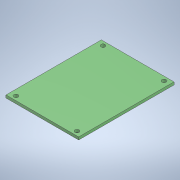
# Autodesk Inventor part: Mock Module PCB
Saved by Autodesk Inventor 2022 (Build 260153000, 153)
## iProperties
Created: 2021-07-19
Part Number: Mock Module PCB
Material: Generic
Document SubType Name: Modeling
Designer: Caleb
Density: 1 g/cm^3
Appearance: Default
Author: Caleb
Autodesk Inventor part; units mm, degrees
ref_plane "YZ Plane" through (0, 0, 0) normal (1, 0, 0) x (0, 1, 0)
ref_plane "XZ Plane" through (0, 0, 0) normal (0, 1, 0) x (-1, 0, 0)
ref_plane "XY Plane" through (0, 0, 0) normal (0, 0, 1) x (1, 0, 0)
sketch "Sketch1" plane through (0, 0, 0) normal (0, 1, 0) x (-1, 0, 0)
  line L0 (-21.5, 28.2) -> (21.5, 28.2)
  line L1 (21.5, 28.2) -> (21.5, -28.2)
  line L2 (21.5, -28.2) -> (-21.5, -28.2)
  line L3 (-21.5, -28.2) -> (-21.5, 28.2)
  line L4 (-21.5, 28.2) -> (21.5, -28.2) construction
  line L5 (21.5, 28.2) -> (-21.5, -28.2) construction
  point P0 (0, 0)
  dimension "d0" = 43
  dimension "d1" = 56.4
  constraints: 12 end point, 2 midpoint, 2 parallel, 1 horizontal, 1 perpendicular
  measures "d0" distance of L0.start L0.end
  measures "d1" distance of L0.end L1.end
extrude "Extrusion1" add sketch "Sketch1" along normal blind 1.6
sketch "Sketch2" plane through (0, 1.6, 0) normal (0, 1, 0) x (1, 0, 0)
  point P0 (0, 0)
  point P1 (-18.05, -25.75)
  point P2 (-18.05, 25.75)
  point P3 (18.05, 25.75)
  point P4 (18.05, -25.75)
  dimension "d19" = 36.1
  dimension "d20" = 51.5
  dimension "d21" = 25.75
  dimension "d22" = 18.05
  constraints: 2 horizontal alignment, 2 vertical alignment
  measures "d19" distance of point (18.05, 25.75) point (-18.05, 25.75)
  measures "d20" distance of point (-18.05, -25.75) point (-18.05, 25.75)
  measures "d21" vertical distance of point (0, 0) point (-18.05, 25.75)
  measures "d22" horizontal distance of point (0, 0) point (18.05, 25.75)
hole "Hole1" at (-18.05, 1.6, 25.75) at (-18.05, 1.6, -25.75) at (18.05, 1.6, -25.75) at (18.05, 1.6, 25.75) direction (0, -1, 0) diameter 2.5 end through all
sketch "Sketch4" plane through (0, 0, 0) normal (0, -1, 0) x (1, 0, 0)
  line L0 (10.5954, -26.3152) -> (-11.3358, -26.3152) construction
  line L1 (-11.3358, -26.3152) -> (-11.3358, -23.0671) construction
  line L2 (-11.3358, -23.0671) -> (10.5954, -23.0671) construction
  line L3 (10.5954, -23.0671) -> (10.5954, -26.3152) construction
  line L4 (7.6734, -23.1313) -> (8.0785, -23.1313)
  line L5 (8.0785, -23.1313) -> (8.0785, -25.7569)
  line L6 (8.0785, -25.7569) -> (8.8738, -23.9711)
  line L7 (8.8738, -23.9711) -> (9.1208, -23.9711)
  line L8 (9.1208, -23.9711) -> (9.9088, -25.7569)
  line L9 (9.9088, -25.7569) -> (9.9088, -23.1313)
  line L10 (9.9088, -23.1313) -> (10.2867, -23.1313)
  line L11 (10.2867, -23.1313) -> (10.2867, -26.1793)
  line L12 (10.2867, -26.1793) -> (9.7334, -26.1793)
  line L13 (9.7334, -26.1793) -> (8.9726, -24.4824)
  line L14 (8.9726, -24.4824) -> (8.2366, -26.1793)
  line L15 (8.2366, -26.1793) -> (7.6734, -26.1793)
  line L16 (7.6734, -26.1793) -> (7.6734, -23.1313)
  spline S0 degree 2 poles (5.2059, -24.2749) (5.2059, -23.6969) (5.7616, -23.0671) (6.226, -23.0671) knots 0 0 0 1 2 2 2
  spline S1 degree 2 poles (6.226, -23.0671) (6.7027, -23.0671) (7.2486, -23.7167) (7.2486, -24.2749) knots 0 0 0 1 2 2 2
  spline S2 degree 2 poles (7.2486, -24.2749) (7.2486, -24.848) (6.6854, -25.4828) (6.226, -25.4828) knots 0 0 0 1 2 2 2
  spline S3 degree 2 poles (6.226, -25.4828) (5.7616, -25.4828) (5.2059, -24.8504) (5.2059, -24.2749) knots 0 0 0 1 2 2 2
  spline S4 degree 2 poles (5.6035, -24.2749) (5.6035, -24.7195) (5.9271, -25.1518) (6.226, -25.1518) knots 0 0 0 1 2 2 2
  spline S5 degree 2 poles (6.226, -25.1518) (6.5249, -25.1518) (6.8509, -24.7195) (6.8509, -24.2749) knots 0 0 0 1 2 2 2
  spline S6 degree 2 poles (6.8509, -24.2749) (6.8509, -23.8427) (6.5249, -23.3981) (6.226, -23.3981) knots 0 0 0 1 2 2 2
  spline S7 degree 2 poles (6.226, -23.3981) (5.9296, -23.3981) (5.6035, -23.8353) (5.6035, -24.2749) knots 0 0 0 1 2 2 2
  line L17 (3.052, -23.1313) -> (3.4373, -23.1313)
  line L18 (3.4373, -23.1313) -> (3.4373, -23.3635)
  spline S8 degree 2 poles (3.4373, -23.3635) (3.5263, -23.2894) (3.6572, -23.1906) (3.7461, -23.1486) knots 0 0 0 1 2 2 2
  spline S9 degree 2 poles (3.7461, -23.1486) (3.8276, -23.1091) (4.003, -23.0671) (4.1191, -23.0671) knots 0 0 0 1 2 2 2
  spline S10 degree 2 poles (4.1191, -23.0671) (4.3068, -23.0671) (4.6229, -23.2227) (4.7341, -23.3734) knots 0 0 0 1 2 2 2
  spline S11 degree 2 poles (4.7341, -23.3734) (4.8452, -23.524) (4.9687, -23.9687) (4.9687, -24.2576) knots 0 0 0 1 2 2 2
  spline S12 degree 2 poles (4.9687, -24.2576) (4.9687, -24.559) (4.8131, -24.9986) (4.6773, -25.1641) knots 0 0 0 1 2 2 2
  spline S13 degree 2 poles (4.6773, -25.1641) (4.5513, -25.3123) (4.1981, -25.4828) (4.003, -25.4828) knots 0 0 0 1 2 2 2
  spline S14 degree 2 poles (4.003, -25.4828) (3.8325, -25.4828) (3.5781, -25.4062) (3.4373, -25.3272) knots 0 0 0 1 2 2 2
  line L19 (3.4373, -25.3272) -> (3.4373, -26.3152)
  line L20 (3.4373, -26.3152) -> (3.052, -26.3152)
  line L21 (3.052, -26.3152) -> (3.052, -23.1313)
  line L22 (3.4373, -23.6871) -> (3.4373, -25.0085)
  spline S15 degree 2 poles (3.4373, -25.0085) (3.5806, -25.0777) (3.8078, -25.1296) (3.9387, -25.1296) knots 0 0 0 1 2 2 2
  spline S16 degree 2 poles (3.9387, -25.1296) (4.2351, -25.1296) (4.5711, -24.685) (4.5711, -24.2651) knots 0 0 0 1 2 2 2
  spline S17 degree 2 poles (4.5711, -24.2651) (4.5711, -23.86) (4.3142, -23.4327) (4.0301, -23.4327) knots 0 0 0 1 2 2 2
  spline S18 degree 2 poles (4.0301, -23.4327) (3.8795, -23.4327) (3.5732, -23.571) (3.4373, -23.6871) knots 0 0 0 1 2 2 2
  line L23 (0.7154, -23.1313) -> (1.1007, -23.1313)
  line L24 (1.1007, -23.1313) -> (1.1007, -23.3833)
  spline S19 degree 2 poles (1.1007, -23.3833) (1.2785, -23.2276) (1.5972, -23.0671) (1.7948, -23.0671) knots 0 0 0 1 2 2 2
  spline S20 degree 2 poles (1.7948, -23.0671) (1.943, -23.0671) (2.2073, -23.1659) (2.3036, -23.2721) knots 0 0 0 1 2 2 2
  spline S21 degree 2 poles (2.3036, -23.2721) (2.4024, -23.3783) (2.5111, -23.7019) (2.5111, -23.9341) knots 0 0 0 1 2 2 2
  line L25 (2.5111, -23.9341) -> (2.5111, -25.4186)
  line L26 (2.5111, -25.4186) -> (2.1258, -25.4186)
  line L27 (2.1258, -25.4186) -> (2.1258, -24.1144)
  spline S22 degree 2 poles (2.1258, -24.1144) (2.1258, -23.9316) (2.0986, -23.692) (2.0517, -23.6031) knots 0 0 0 1 2 2 2
  spline S23 degree 2 poles (2.0517, -23.6031) (2.0047, -23.5142) (1.8442, -23.4327) (1.6935, -23.4327) knots 0 0 0 1 2 2 2
  spline S24 degree 2 poles (1.6935, -23.4327) (1.5527, -23.4327) (1.2341, -23.5932) (1.1007, -23.7093) knots 0 0 0 1 2 2 2
  line L28 (1.1007, -23.7093) -> (1.1007, -25.4186)
  line L29 (1.1007, -25.4186) -> (0.7154, -25.4186)
  line L30 (0.7154, -25.4186) -> (0.7154, -23.1313)
  line L31 (-0.2356, -23.1313) -> (0.1497, -23.1313)
  line L32 (0.1497, -23.1313) -> (0.1497, -26.3152)
  line L33 (0.1497, -26.3152) -> (-0.2356, -26.3152)
  line L34 (-0.2356, -26.3152) -> (-0.2356, -23.1313)
  spline S25 degree 2 poles (-1.7942, -23.0794) (-1.2458, -23.0794) (-0.6431, -23.6945) (-0.6431, -24.2626) knots 0 0 0 1 2 2 2
  spline S26 degree 2 poles (-0.6431, -24.2626) (-0.6431, -24.8208) (-1.2285, -25.4828) (-1.7003, -25.4828) knots 0 0 0 1 2 2 2
  spline S27 degree 2 poles (-1.7003, -25.4828) (-1.9127, -25.4828) (-2.2412, -25.3593) (-2.3623, -25.2284) knots 0 0 0 1 2 2 2
  spline S28 degree 2 poles (-2.3623, -25.2284) (-2.4858, -25.0974) (-2.6167, -24.7195) (-2.6167, -24.4454) knots 0 0 0 1 2 2 2
  line L35 (-2.6167, -24.4454) -> (-2.6167, -24.2354)
  line L36 (-2.6167, -24.2354) -> (-1.0334, -24.2354)
  spline S29 degree 2 poles (-1.0334, -24.2354) (-1.0334, -23.8377) (-1.4335, -23.4154) (-1.7892, -23.4154) knots 0 0 0 1 2 2 2
  spline S30 degree 2 poles (-1.7892, -23.4154) (-1.9152, -23.4154) (-2.1597, -23.4722) (-2.2585, -23.5166) knots 0 0 0 1 2 2 2
  spline S31 degree 2 poles (-2.2585, -23.5166) (-2.3623, -23.566) (-2.5055, -23.6525) (-2.5525, -23.692) knots 0 0 0 1 2 2 2
  line L37 (-2.5525, -23.692) -> (-2.5747, -23.692)
  line L38 (-2.5747, -23.692) -> (-2.5747, -23.2721)
  spline S32 degree 2 poles (-2.5747, -23.2721) (-2.508, -23.2449) (-2.3055, -23.1659) (-2.2264, -23.1437) knots 0 0 0 1 2 2 2
  spline S33 degree 2 poles (-2.2264, -23.1437) (-2.1153, -23.1116) (-1.9325, -23.0794) (-1.7942, -23.0794) knots 0 0 0 1 2 2 2
  spline S34 degree 2 poles (-2.2412, -24.5293) (-2.2363, -24.685) (-2.1721, -24.9122) (-2.1103, -24.9888) knots 0 0 0 1 2 2 2
  spline S35 degree 2 poles (-2.1103, -24.9888) (-2.0436, -25.0752) (-1.8337, -25.1666) (-1.6781, -25.1666) knots 0 0 0 1 2 2 2
  spline S36 degree 2 poles (-1.6781, -25.1666) (-1.5249, -25.1666) (-1.31, -25.0752) (-1.2211, -24.9863) knots 0 0 0 1 2 2 2
  spline S37 degree 2 poles (-1.2211, -24.9863) (-1.1347, -24.8949) (-1.0457, -24.6751) (-1.0334, -24.5293) knots 0 0 0 1 2 2 2
  line L39 (-1.0334, -24.5293) -> (-2.2412, -24.5293)
  spline S38 degree 2 poles (-6.2723, -25.2605) (-6.2723, -25.0629) (-6.1315, -24.7072) (-6.0055, -24.5837) knots 0 0 0 1 2 2 2
  spline S39 degree 2 poles (-6.0055, -24.5837) (-5.8475, -24.4281) (-5.4201, -24.2675) (-5.0941, -24.2675) knots 0 0 0 1 2 2 2
  line L40 (-5.0941, -24.2675) -> (-4.7508, -24.2675)
  line L41 (-4.7508, -24.2675) -> (-4.7508, -23.1313)
  line L42 (-4.7508, -23.1313) -> (-4.3457, -23.1313)
  line L43 (-4.3457, -23.1313) -> (-4.3457, -26.1793)
  line L44 (-4.3457, -26.1793) -> (-5.1114, -26.1793)
  spline S40 degree 2 poles (-5.1114, -26.1793) (-5.3831, -26.1793) (-5.7635, -26.0904) (-5.9092, -25.9891) knots 0 0 0 1 2 2 2
  spline S41 degree 2 poles (-5.9092, -25.9891) (-6.0796, -25.873) (-6.2723, -25.5149) (-6.2723, -25.2605) knots 0 0 0 1 2 2 2
  spline S42 degree 2 poles (-5.8499, -25.2481) (-5.8499, -25.4062) (-5.7412, -25.6384) (-5.6301, -25.7125) knots 0 0 0 1 2 2 2
  spline S43 degree 2 poles (-5.6301, -25.7125) (-5.5338, -25.7767) (-5.2769, -25.8286) (-5.0867, -25.8286) knots 0 0 0 1 2 2 2
  line L45 (-5.0867, -25.8286) -> (-4.7508, -25.8286)
  line L46 (-4.7508, -25.8286) -> (-4.7508, -24.6133)
  line L47 (-4.7508, -24.6133) -> (-5.0274, -24.6133)
  spline S44 degree 2 poles (-5.0274, -24.6133) (-5.2744, -24.6133) (-5.5782, -24.6924) (-5.677, -24.7961) knots 0 0 0 1 2 2 2
  spline S45 degree 2 poles (-5.677, -24.7961) (-5.7684, -24.8875) (-5.8499, -25.1024) (-5.8499, -25.2481) knots 0 0 0 1 2 2 2
  spline S46 degree 2 poles (-7.8482, -23.077) (-7.5518, -23.077) (-7.0504, -23.277) (-6.8676, -23.4771) knots 0 0 0 1 2 2 2
  spline S47 degree 2 poles (-6.8676, -23.4771) (-6.6848, -23.6747) (-6.4847, -24.2675) (-6.4847, -24.6528) knots 0 0 0 1 2 2 2
  spline S48 degree 2 poles (-6.4847, -24.6528) (-6.4847, -25.0357) (-6.6799, -25.6038) (-6.8651, -25.8138) knots 0 0 0 1 2 2 2
  spline S49 degree 2 poles (-6.8651, -25.8138) (-7.0479, -26.0188) (-7.5468, -26.2337) (-7.8556, -26.2337) knots 0 0 0 1 2 2 2
  spline S50 degree 2 poles (-7.8556, -26.2337) (-8.0087, -26.2337) (-8.278, -26.1892) (-8.3916, -26.1546) knots 0 0 0 1 2 2 2
  spline S51 degree 2 poles (-8.3916, -26.1546) (-8.4904, -26.1225) (-8.6954, -26.0311) (-8.7967, -25.9768) knots 0 0 0 1 2 2 2
  line L48 (-8.7967, -25.9768) -> (-8.7967, -25.4877)
  line L49 (-8.7967, -25.4877) -> (-8.7645, -25.4877)
  spline S52 degree 2 poles (-8.7645, -25.4877) (-8.7102, -25.5371) (-8.5422, -25.6754) (-8.4212, -25.7421) knots 0 0 0 1 2 2 2
  spline S53 degree 2 poles (-8.4212, -25.7421) (-8.3051, -25.8063) (-8.031, -25.8879) (-7.8531, -25.8879) knots 0 0 0 1 2 2 2
  spline S54 degree 2 poles (-7.8531, -25.8879) (-7.658, -25.8879) (-7.3097, -25.7273) (-7.1788, -25.5742) knots 0 0 0 1 2 2 2
  spline S55 degree 2 poles (-7.1788, -25.5742) (-7.0504, -25.4186) (-6.9071, -24.9468) (-6.9071, -24.6528) knots 0 0 0 1 2 2 2
  spline S56 degree 2 poles (-6.9071, -24.6528) (-6.9071, -24.3392) (-7.0578, -23.8871) (-7.1887, -23.7315) knots 0 0 0 1 2 2 2
  spline S57 degree 2 poles (-7.1887, -23.7315) (-7.3171, -23.5809) (-7.6605, -23.4277) (-7.8531, -23.4277) knots 0 0 0 1 2 2 2
  spline S58 degree 2 poles (-7.8531, -23.4277) (-8.0285, -23.4277) (-8.3274, -23.5142) (-8.4434, -23.5784) knots 0 0 0 1 2 2 2
  spline S59 degree 2 poles (-8.4434, -23.5784) (-8.5546, -23.6426) (-8.7201, -23.776) (-8.767, -23.8229) knots 0 0 0 1 2 2 2
  line L50 (-8.767, -23.8229) -> (-8.7967, -23.8229)
  line L51 (-8.7967, -23.8229) -> (-8.7967, -23.3388)
  spline S60 degree 2 poles (-8.7967, -23.3388) (-8.6954, -23.2919) (-8.5175, -23.2054) (-8.3916, -23.1659) knots 0 0 0 1 2 2 2
  spline S61 degree 2 poles (-8.3916, -23.1659) (-8.2582, -23.1214) (-8.031, -23.077) (-7.8482, -23.077) knots 0 0 0 1 2 2 2
  spline S62 degree 2 poles (-11.242, -24.0675) (-11.242, -23.8402) (-11.0691, -23.4919) (-10.9258, -23.3783) knots 0 0 0 1 2 2 2
  spline S63 degree 2 poles (-10.9258, -23.3783) (-10.7529, -23.2449) (-10.3602, -23.1313) (-10.049, -23.1313) knots 0 0 0 1 2 2 2
  line L52 (-10.049, -23.1313) -> (-9.1746, -23.1313)
  line L53 (-9.1746, -23.1313) -> (-9.1746, -26.1793)
  line L54 (-9.1746, -26.1793) -> (-9.9823, -26.1793)
  spline S64 degree 2 poles (-9.9823, -26.1793) (-10.3083, -26.1793) (-10.6344, -26.1373) (-10.7826, -26.0558) knots 0 0 0 1 2 2 2
  spline S65 degree 2 poles (-10.7826, -26.0558) (-10.948, -25.9694) (-11.0987, -25.6853) (-11.0987, -25.4927) knots 0 0 0 1 2 2 2
  spline S66 degree 2 poles (-11.0987, -25.4927) (-11.0987, -25.2778) (-10.8715, -24.9369) (-10.6714, -24.8406) knots 0 0 0 1 2 2 2
  line L55 (-10.6714, -24.8406) -> (-10.6714, -24.8257)
  spline S67 degree 2 poles (-10.6714, -24.8257) (-10.9431, -24.7516) (-11.242, -24.3589) (-11.242, -24.0675) knots 0 0 0 1 2 2 2
  spline S68 degree 2 poles (-10.8196, -24.0502) (-10.8196, -24.2231) (-10.7208, -24.4454) (-10.5726, -24.5244) knots 0 0 0 1 2 2 2
  spline S69 degree 2 poles (-10.5726, -24.5244) (-10.4763, -24.5738) (-10.249, -24.6034) (-10.0391, -24.6034) knots 0 0 0 1 2 2 2
  line L56 (-10.0391, -24.6034) -> (-9.5797, -24.6034)
  line L57 (-9.5797, -24.6034) -> (-9.5797, -23.4771)
  line L58 (-9.5797, -23.4771) -> (-9.9082, -23.4771)
  spline S70 degree 2 poles (-9.9082, -23.4771) (-10.1749, -23.4771) (-10.4812, -23.5265) (-10.5998, -23.6056) knots 0 0 0 1 2 2 2
  spline S71 degree 2 poles (-10.5998, -23.6056) (-10.7134, -23.6871) (-10.8196, -23.8896) (-10.8196, -24.0502) knots 0 0 0 1 2 2 2
  spline S72 degree 2 poles (-10.6763, -25.4358) (-10.6763, -25.5445) (-10.6022, -25.7075) (-10.5207, -25.7545) knots 0 0 0 1 2 2 2
  spline S73 degree 2 poles (-10.5207, -25.7545) (-10.4219, -25.8088) (-10.1823, -25.8335) (-9.9674, -25.8335) knots 0 0 0 1 2 2 2
  line L59 (-9.9674, -25.8335) -> (-9.5797, -25.8335)
  line L60 (-9.5797, -25.8335) -> (-9.5797, -24.9418)
  line L61 (-9.5797, -24.9418) -> (-10.0391, -24.9418)
  spline S74 degree 2 poles (-10.0391, -24.9418) (-10.2293, -24.9418) (-10.4096, -24.9814) (-10.5059, -25.0431) knots 0 0 0 1 2 2 2
  spline S75 degree 2 poles (-10.5059, -25.0431) (-10.5998, -25.1024) (-10.6763, -25.2926) (-10.6763, -25.4358) knots 0 0 0 1 2 2 2
  point P0 (0, 0)
  constraints: 2 other
emboss "Emboss2" sketch "Sketch4" operation add depth 0.05 direction (0, 1, 0)
body "Solid1"
